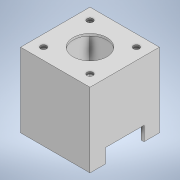
# Autodesk Inventor part: Корпус для двигателя
Saved by Autodesk Inventor 2021 (Build 250183000, 183)
## iProperties
Created: 2021-08-05
Part Number: Корпус для двигателя
Material: Типовые
Document SubType Name: Modeling
Designer: User
Density: 1 g/cm^3
Appearance: По умолчанию
Author: User
Autodesk Inventor part; units mm, degrees
ref_plane "YZ Plane" through (0, 0, 0) normal (1, 0, 0) x (0, 1, 0)
ref_plane "XZ Plane" through (0, 0, 0) normal (0, 1, 0) x (-1, 0, 0)
ref_plane "XY Plane" through (0, 0, 0) normal (0, 0, 1) x (1, 0, 0)
sketch "Эскиз1" plane through (0, 0, 0) normal (0, 1, 0) x (-1, 0, 0)
  line L0 (-21.15, 21.15) -> (21.15, 21.15)
  line L1 (21.15, 21.15) -> (21.15, -21.15)
  line L2 (21.15, -21.15) -> (-21.15, -21.15)
  line L3 (-21.15, -21.15) -> (-21.15, 21.15)
  line L4 (-21.15, 21.15) -> (21.15, -21.15) construction
  line L5 (21.15, 21.15) -> (-21.15, -21.15) construction
  line L6 (-23.15, 23.15) -> (23.15, 23.15)
  line L7 (23.15, 23.15) -> (23.15, -23.15)
  line L8 (23.15, -23.15) -> (-23.15, -23.15)
  line L9 (-23.15, -23.15) -> (-23.15, 23.15)
  line L10 (-23.15, 23.15) -> (23.15, -23.15) construction
  line L11 (23.15, 23.15) -> (-23.15, -23.15) construction
  point P0 (0, 0)
  dimension "d0" = 42.3
  dimension "d1" = 42.3
  dimension "d2" = 46.3
  dimension "d3" = 46.3
  constraints: 24 end point, 4 midpoint, 4 parallel, 2 horizontal, 2 perpendicular
  measures "d0" distance of L1.end L2.end
  measures "d1" distance of L0.end L1.end
  measures "d2" distance of L7.end L8.end
  measures "d3" distance of L6.end L7.end
extrude "Выдавливание1" add sketch "Эскиз1" along normal blind 48
sketch "Эскиз2" plane through (23.15, 0, 23.15) normal (1, 0, 0) x (0, 0, -1)
  line L0 (23.15, 9.5) -> (36.05, 9.5)
  line L1 (36.05, 9.5) -> (10.25, 9.5)
  line L2 (10.25, 9.5) -> (10.25, 0)
  line L3 (44.3, 0) -> (2, 0) projected
  line L4 (36.05, 9.5) -> (36.05, 0)
  point P0 (23.15, 0)
  dimension "d6" = 9.5
  dimension "d7" = 12.9
  dimension "d8" = 25.8
  constraints: 8 end point, 2 point on line, 1 perpendicular, 1 vertical
  measures "d6" distance of point (23.15, 0) L0.start
  measures "d7" distance of L0.start L0.end
  measures "d8" distance of L0.end L1.end
extrude "Выдавливание2" cut sketch "Эскиз2" against normal blind 2
sketch "Эскиз3" plane through (0, 48, 0) normal (0, 1, 0) x (1, 0, 0)
  line L0 (-23.15, 23.15) -> (-23.15, -23.15) projected
  line L1 (23.15, -23.15) -> (-23.15, -23.15)
  line L2 (-23.15, -23.15) -> (-23.15, 23.15)
  line L3 (-23.15, 23.15) -> (23.15, 23.15)
  line L4 (23.15, 23.15) -> (23.15, -23.15)
  line L5 (23.15, -23.15) -> (-23.15, 23.15) construction
  line L6 (-23.15, -23.15) -> (23.15, 23.15) construction
  point P0 (0, 0)
  constraints: 12 end point, 2 midpoint, 2 parallel, 1 horizontal, 1 perpendicular
extrude "Выдавливание3" add sketch "Эскиз3" along normal blind 1.5
sketch "Эскиз4" plane through (0, 49.5, 0) normal (0, 1, 0) x (1, 0, 0)
  circle A0 centre (0, 0) radius 11.25
  line L0 (15.5, 15.5) -> (-15.5, 15.5)
  line L1 (-15.5, 15.5) -> (-15.5, -15.5)
  line L2 (-15.5, -15.5) -> (15.5, -15.5)
  line L3 (15.5, -15.5) -> (15.5, 15.5)
  line L4 (15.5, 15.5) -> (-15.5, -15.5) construction
  line L5 (-15.5, 15.5) -> (15.5, -15.5) construction
  circle A1 centre (-15.5, -15.5) radius 2
  circle A2 centre (-15.5, 15.5) radius 2
  circle A3 centre (15.5, 15.5) radius 2
  circle A4 centre (15.5, -15.5) radius 2
  dimension "d13" = 22.5
  dimension "d14" = 31
  dimension "d15" = 31
  dimension "d16" = 4
  dimension "d17" = 4
  dimension "d18" = 4
  dimension "d19" = 4
  constraints: 12 end point, 5 centre point, 5 coincident, 2 midpoint, 2 parallel, 1 horizontal, 1 perpendicular
  measures "d13" diameter of A0
  measures "d14" distance of L2.end L1.end
  measures "d15" distance of L1.end L0.end
  measures "d16" diameter of A1
  measures "d17" diameter of A2
  measures "d18" diameter of A3
  measures "d19" diameter of A4
extrude "Выдавливание4" cut sketch "Эскиз4" against normal blind 1.5 contours A0 | A2 L1 L0 | L0 L1 A2 | A3 L3 L0 | L0 L3 A3 | A1 L2 L1 | L1 L2 A1 | A4 L2 L3 | L3 L2 A4
